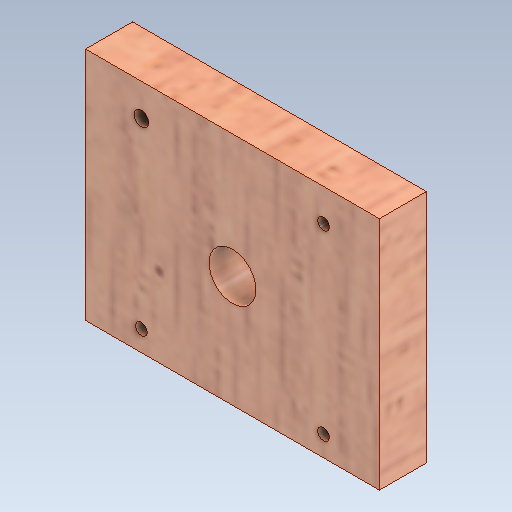
# Autodesk Inventor part: 0005-10-020 suport motor y
Saved by Autodesk Inventor 2020 (Build 240168000, 168)
## iProperties
Created: 2020-12-18
Part Number: 0005-10-020 suport motor y
Material: Generic
Document SubType Name: Modeling
Designer: Iulian Bors
Density: 1 g/cm^3
Appearance: White Oak - Natural Medium Gloss
Author: Iulian Bors
Subject: 020
Autodesk Inventor part; units mm, degrees
ref_plane "YZ Plane" through (0, 0, 0) normal (1, 0, 0) x (0, 1, 0)
ref_plane "XZ Plane" through (0, 0, 0) normal (0, 1, 0) x (-1, 0, 0)
ref_plane "XY Plane" through (0, 0, 0) normal (0, 0, 1) x (1, 0, 0)
sketch "Sketch1" plane through (0, 0, 0) normal (0, 0, 1) x (1, 0, 0)
  line L0 (-25, 20) -> (25, 20)
  line L1 (25, 20) -> (25, -20)
  line L2 (25, -20) -> (-25, -20)
  line L3 (-25, -20) -> (-25, 20)
  point P0 (0, 0)
  point P1 (0, 20)
  point P2 (-25, 0)
  dimension "d0" = 50
  dimension "d1" = 40
  constraints: 8 end point, 2 midpoint, 2 parallel, 1 horizontal, 1 horizontal alignment, 1 perpendicular, 1 vertical alignment
  measures "d0" distance of L0.start L0.end
  measures "d1" distance of L2.end L0.start
extrude "Extrusion1" add sketch "Sketch1" along normal blind 8
sketch "Sketch5" plane through (0, 0, 0) normal (0, 0, -1) x (-1, 0, 0)
  circle A0 centre (-15.5, -16.5) radius 1 projected
  circle A1 centre (15.5, -16.5) radius 1 projected
  circle A2 centre (-15.5, 14.5) radius 1 projected
  circle A3 centre (15.5, 14.5) radius 1.25 projected
  arc A4 (-2, -2.5) -> (-2, 0.5) centre (0, -1) ccw
  line L0 (-2, -2.5) -> (-2, 0.5)
  circle A5 centre (0, -1) radius 4
  point P0 (0, 0)
  dimension "d29" = 8
  constraints: 2 centre point, 2 end point, 2 point on circle, 1 coincident, 1 vertical, 4 other
  measures "d29" diameter of A5
extrude "Extrusion5" cut sketch "Sketch5" against normal through all contours A0 | A1 | A2 | A3 | L0 A4 | A5
body "Solid1"
